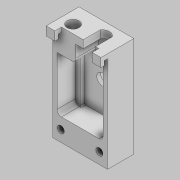
# Autodesk Inventor part: case
Saved by Autodesk Inventor 2021.4 (Build 254397000, 397)
## iProperties
Created: 2022-10-31
Part Number: case
Material: Generisch
Document SubType Name: Modeling
Designer: Tilman Preuschoff
Density: 1 g/cm^3
Appearance: Vorgabe
Author: Tilman Preuschoff
Autodesk Inventor part; units mm, degrees
ref_plane "YZ Plane" through (0, 0, 0) normal (1, 0, 0) x (0, 1, 0)
ref_plane "XZ Plane" through (0, 0, 0) normal (0, 1, 0) x (-1, 0, 0)
ref_plane "XY Plane" through (0, 0, 0) normal (0, 0, 1) x (1, 0, 0)
sketch "Skizze1" plane through (0, 0, 0) normal (0, 0, 1) x (1, 0, 0)
  line L0 (-12.5, 22.5) -> (12.5, 22.5)
  line L1 (12.5, 22.5) -> (12.5, -22.5)
  line L2 (12.5, -22.5) -> (-12.5, -22.5)
  line L3 (-12.5, -22.5) -> (-12.5, 22.5)
  line L4 (-12.5, 22.5) -> (12.5, -22.5) construction
  line L5 (12.5, 22.5) -> (-12.5, -22.5) construction
  point P0 (0, 0)
  dimension "d0" = 25
  dimension "d1" = 45
  constraints: 12 end point, 2 midpoint, 2 parallel, 1 horizontal, 1 perpendicular
  measures "d0" distance between parallel lines of L1 L3
  measures "d1" distance between parallel lines of L0 L2
extrude "Extrusion1" add sketch "Skizze1" along normal blind 12
sketch "Skizze2" plane through (0, 0, 12) normal (0, 0, 1) x (1, 0, 0)
  line L0 (-8.5, 19) -> (8.5, 19)
  line L1 (10.5, 17) -> (10.5, -11)
  line L2 (8.5, -13) -> (-8.5, -13)
  line L3 (-10.5, -11) -> (-10.5, 17)
  line L4 (-10.5, 19) -> (10.5, -13) construction
  line L5 (10.5, 19) -> (-10.5, -13) construction
  line L6 (12.5, 22.5) -> (-12.5, 22.5) projected
  arc A0 (-8.5, 19) -> (-10.5, 17) centre (-8.5, 17) ccw
  arc A1 (10.5, 17) -> (8.5, 19) centre (8.5, 17) ccw
  arc A2 (8.5, -13) -> (10.5, -11) centre (8.5, -11) ccw
  arc A3 (-10.5, -11) -> (-8.5, -13) centre (-8.5, -11) ccw
  point P0 (0, 0)
  point P1 (0, 3)
  point P2 (0, 3)
  dimension "d4" = 21
  dimension "d5" = 3.5
  dimension "d6" = 32
  dimension "d7" = 2
  constraints: 12 end point, 8 point on circle, 8 point on line, 8 tangent, 4 centre point, 3 equal radius, 3 midpoint, 2 parallel, 1 horizontal, 1 perpendicular, 1 vertical alignment
  measures "d4" distance between parallel lines of L1 L3
  measures "d5" distance between parallel lines of L6 L0
  measures "d6" distance between parallel lines of L2 L0
  measures "d7" radius of A0
extrude "Extrusion2" cut sketch "Skizze2" against normal blind 8.2
sketch "Skizze4" plane through (0, 0, 3.8) normal (0, 0, 1) x (1, 0, 0)
  line L0 (-12.5, -22.5) -> (12.5, -22.5) projected
  point P0 (0, 0)
  point P1 (0, 1)
  dimension "d79" = 23.5
  constraints: 1 vertical alignment
  measures "d79" distance from line of L0 point (0, 1)
hole "Bohrung2" at (0, 1, 3.8) direction (0, 0, -1) diameter 5.2 end through all
sketch "Skizze5" plane through (0, 0, 3.8) normal (0, 0, 1) x (1, 0, 0)
  line L0 (-8.5, 19) -> (8.5, 19) projected
  line L1 (-7.7, 19) -> (6.95, 19)
  line L2 (8.2, 21) -> (8.2, -12.5)
  line L3 (7.7, -13) -> (-7.7, -13)
  line L4 (-8.2, -12.5) -> (-8.2, 18.5)
  arc A0 (-7.7, 19) -> (-8.2, 18.5) centre (-7.7, 18.5) ccw
  arc A1 (7.7, -13) -> (8.2, -12.5) centre (7.7, -12.5) ccw
  arc A2 (-8.2, -12.5) -> (-7.7, -13) centre (-7.7, -12.5) ccw
  line L5 (10.5, 17) -> (10.5, -11) projected
  line L6 (6.95, 19) -> (7.7, 19)
  line L7 (8.2, 21) -> (8.2, 18.5)
  arc A3 (8.2, 18.5) -> (7.7, 19) centre (7.7, 18.5) ccw
  line L8 (-10.5, -11) -> (-10.5, 17) projected
  line L9 (8.5, -13) -> (-8.5, -13) projected
  point P0 (0, 0)
  point P1 (-8.2, 19)
  point P2 (8.2, 19)
  point P3 (8.2, 18.5)
  point P4 (4, -13)
  point P5 (7.7, -13)
  point P6 (6.2, 19)
  dimension "d28" = 0.5
  dimension "d29" = 2.3
  dimension "d39" = 0.5
  dimension "d67" = 0.5
  dimension "d73" = 2.3
  constraints: 12 end point, 8 point on circle, 8 tangent, 7 point on line, 4 centre point, 2 parallel, 2 perpendicular, 1 equal radius, 1 horizontal, 1 horizontal alignment
  measures "d28" radius of A0
  measures "d29" distance between parallel lines of L5 L2
  measures "d39" radius of A3
  measures "d67" radius of A1
  measures "d73" distance between parallel lines of L8 L4
sketch "Skizze6" plane through (0, 0, 12) normal (0, 0, 1) x (1, 0, 0)
  line L0 (12.5, 22.5) -> (-12.5, 22.5) projected
  line L1 (-8.5, 19) -> (8.5, 19) projected
  line L2 (-1.1, 22.5) -> (5.9, 22.5)
  line L3 (5.9, 22.5) -> (5.9, 19)
  line L4 (5.9, 19) -> (-1.1, 19)
  line L5 (-1.1, 19) -> (-1.1, 22.5)
  line L6 (12.5, -22.5) -> (12.5, 22.5) projected
  line L7 (7.95, 22) -> (7.95, 17) projected
  point P0 (0, 0)
  point P1 (6.95, 22)
  point P2 (8.5, 19)
  point P3 (5.9, 20.75)
  point P4 (7.95, 19.5)
  dimension "d34" = 7
  dimension "d38" = 6.6
  constraints: 8 end point, 2 midpoint, 2 parallel, 1 horizontal, 1 perpendicular, 1 point on line, 2 other
  measures "d34" distance between parallel lines of L3 L5
  measures "d38" distance between parallel lines of L6 L3
extrude "Extrusion4" [suppressed]
extrude "Extrusion5" cut sketch "Skizze5" against normal blind 2 contours L0 A3 L2 A1 L3 A2 L4 A0
sketch "Skizze7" plane through (-12.5, -22.5, 0) normal (0, -1, 0) x (1, 0, 0)
  line L0 (0, 0) -> (25, 0) projected
  point P0 (12.5, 0)
  point P1 (12.5, 7)
  point P2 (12.5, 0)
  dimension "d42" = 7
  constraints: 1 midpoint, 1 vertical alignment
  measures "d42" distance from line of point (12.5, 7) L0
hole "Bohrung3" at (0, -22.5, 7) direction (0, 1, 0) diameter 5.6 depth 8
sketch "Skizze11" plane through (-12.5, 22.5, 0) normal (0, 1, 0) x (1, 0, 0)
  line L0 (4, -12) -> (21, -12) projected
  line L1 (13.95, -12) -> (19.45, -12)
  line L2 (19.45, -12) -> (19.45, -4)
  line L3 (19.45, -4) -> (13.95, -4)
  line L4 (13.95, -4) -> (13.95, -12)
  line L5 (25, 0) -> (25, -12) projected
  line L6 (25, 0) -> (0, 0) projected
  circle A0 centre (16.7, -6.1) radius 3.3
  point P0 (12.5, 0)
  point P1 (7.5, -12)
  point P2 (16.7, -4)
  point P3 (19.45, -4.2759)
  point P4 (13.95, -4.2759)
  dimension "d68" = 5.5
  dimension "d69" = 5.55
  dimension "d91" = 6.6
  dimension "d92" = 6.1
  dimension "d93" = 8
  constraints: 8 end point, 2 parallel, 1 centre point, 1 horizontal, 1 midpoint, 1 perpendicular, 1 point on line, 1 vertical alignment
  measures "d68" distance between parallel lines of L2 L4
  measures "d69" distance between parallel lines of L5 L2
  measures "d91" diameter of A0
  measures "d92" distance from line of L6 A0.centre
  measures "d93" distance between parallel lines of L3 L0
extrude "Extrusion8" cut sketch "Skizze11" against normal up to surface (3.5 mm away) contours L4 A0 L2 L0 | L4 A0 L3 L2 | A0 L3
sketch "Skizze13" plane through (0, 0, 12) normal (0, 0, 1) x (1, 0, 0)
  line L0 (12.5, 22.5) -> (-12.5, 22.5) projected
  line L1 (-12.5, 22.5) -> (-2, 22.5)
  line L2 (-2, 22.5) -> (-2, 13.5)
  line L3 (-4, 11.5) -> (-12.5, 11.5)
  line L4 (-12.5, 11.5) -> (-12.5, 22.5)
  arc A0 (-4, 11.5) -> (-2, 13.5) centre (-4, 13.5) ccw
  point P0 (0, 0)
  dimension "d94" = 2
  dimension "d95" = 10.5
  dimension "d96" = 11
  constraints: 8 end point, 2 parallel, 2 point on circle, 2 tangent, 1 centre point, 1 horizontal, 1 perpendicular
  measures "d94" radius of A0
  measures "d95" distance between parallel lines of L4 L2
  measures "d96" distance from line of L1.end L3
extrude "Extrusion9" add sketch "Skizze13" against normal up to surface (12 mm away)
sketch "Skizze14" plane through (-12.5, 22.5, 0) normal (0, 1, 0) x (1, 0, 0)
  circle A0 centre (5.5, -8.25) radius 2.75
  line L0 (2, -3.8) -> (2, -12) projected
  line L1 (25, 0) -> (0, 0) projected
  line L2 (0, 0) -> (0, -12) projected
  point P0 (12.5, 0)
  point P1 (12.9295, 0.3417)
  point P2 (1.9355, -9.867)
  dimension "d101" = 5.5
  dimension "d102" = 8.25
  dimension "d114" = 5.5
  constraints: 1 centre point
  measures "d101" diameter of A0
  measures "d102" distance from line of L1 A0.centre
  measures "d114" distance from line of A0.centre L2
extrude "Extrusion10" cut sketch "Skizze14" against normal up to surface (11 mm away)
sketch "Skizze15" plane through (0, 0, 0) normal (0, 0, -1) x (-1, 0, 0)
  line L0 (-12.5, 22.5) -> (12.5, 22.5) projected
  line L1 (12.5, 22.5) -> (12.5, -22.5) projected
  point P0 (0, 0)
  point P1 (7, 16.5)
  point P2 (0, 0)
  dimension "d112" = 6
  dimension "d113" = 5.5
  constraints: 1 coincident
  measures "d112" distance from line of point (7, 16.5) L0
  measures "d113" distance from line of point (7, 16.5) L1
hole "Bohrung6" at (-7, 16.5, 0) direction (0, 0, 1) diameter 5.6 depth 8
sketch "Skizze20" plane through (-12.5, -22.5, 0) normal (0, -1, 0) x (1, 0, 0)
  line L0 (0, 12) -> (0.7, 12) projected
  line L1 (0, 0) -> (25, 0) projected
  line L2 (0, 12) -> (25, 12)
  line L3 (25, 12) -> (25, 0)
  line L4 (25, 0) -> (0, 0)
  line L5 (0, 0) -> (0, 12)
  circle A0 centre (12.5, 7) radius 2.8 projected
  circle A1 centre (12.5, 7) radius 2.8
  point P0 (12.5, 0)
  constraints: 8 end point, 2 parallel, 1 centre point, 1 coincident, 1 horizontal, 1 perpendicular
extrude "Extrusion15" add sketch "Skizze20" along normal blind 0.7
sketch "Skizze21" plane through (0, 0, 12) normal (0, 0, 1) x (1, 0, 0)
  line L0 (-12.5, 22.5) -> (-12.5, -23.2) projected
  line L1 (-12.5, 22.5) -> (-8.5, 22.5)
  line L2 (-8.5, 22.5) -> (-8.5, 20.5)
  line L3 (-8.5, 20.5) -> (-12.5, 20.5)
  line L4 (-12.5, 20.5) -> (-12.5, 22.5)
  line L5 (12.5, 22.5) -> (12.5, -23.2) projected
  line L6 (12.5, 22.5) -> (8.5, 22.5)
  line L7 (8.5, 22.5) -> (8.5, 20.5)
  line L8 (8.5, 20.5) -> (12.5, 20.5)
  line L9 (12.5, 20.5) -> (12.5, 22.5)
  point P0 (0, 0)
  dimension "d139" = 2
  dimension "d140" = 2
  dimension "d141" = 4
  dimension "d142" = 4
  constraints: 16 end point, 4 parallel, 2 horizontal, 2 perpendicular
  measures "d139" distance between parallel lines of L6 L8
  measures "d140" distance between parallel lines of L1 L3
  measures "d141" distance between parallel lines of L5 L7
  measures "d142" distance between parallel lines of L0 L2
extrude "Extrusion16" add sketch "Skizze21" along normal blind 1.5
sketch "Skizze22" plane through (0, 0, 13.5) normal (0, 0, 1) x (1, 0, 0)
  line L0 (-12.5, 22.5) -> (-12.5, -23.2) projected
  line L1 (8.5, 20.5) -> (8.5, 22.5) projected
  line L2 (12.5, 20.5) -> (12.5, -23.2) projected
  line L3 (8.5, 22.5) -> (12.5, 22.5)
  line L4 (12.5, 22.5) -> (12.5, 18.5)
  line L5 (12.5, 18.5) -> (8.5, 18.5)
  line L6 (8.5, 18.5) -> (8.5, 22.5)
  line L7 (-8.5, 22.5) -> (-8.5, 20.5) projected
  line L8 (-12.5, 20.5) -> (-12.5, -23.2) projected
  line L9 (-8.5, 22.5) -> (-12.5, 22.5)
  line L10 (-12.5, 22.5) -> (-12.5, 18.5)
  line L11 (-12.5, 18.5) -> (-8.5, 18.5)
  line L12 (-8.5, 18.5) -> (-8.5, 22.5)
  point P0 (0, 0)
  dimension "d145" = 4
  dimension "d146" = 4
  constraints: 16 end point, 4 parallel, 2 horizontal, 2 perpendicular, 2 point on line
  measures "d145" distance between parallel lines of L9 L11
  measures "d146" distance between parallel lines of L3 L5
extrude "Extrusion17" add sketch "Skizze22" along normal blind 1.5
sketch "Skizze23" plane through (0, 0, 12) normal (0, 0, 1) x (1, 0, 0)
  line L0 (-8.8, -18.1) -> (8.8, -18.1)
  line L1 (-12.5, 20.5) -> (-12.5, -23.2) projected
  line L2 (12.5, 20.5) -> (12.5, -23.2) projected
  line L3 (8.5, -13) -> (-8.5, -13) projected
  line L4 (12.5, -23.2) -> (-12.5, -23.2) projected
  point P0 (0, 0)
  dimension "d149" = 3.7
  dimension "d150" = 3.7
  dimension "d152" = 5.1
  dimension "d153" = 10.2
  constraints: 2 end point, 1 horizontal
  measures "d149" distance from line of L1 L0.start
  measures "d150" distance from line of L2 L0.end
  measures "d152" distance between parallel lines of L4 L0
  measures "d153" distance between parallel lines of L4 L3
hole "Bohrung7" at (-8.8, -18.1, 12) at (8.8, -18.1, 12) direction (0, 0, -1) diameter 3.2 depth 8
equation "\"d152\" = 0.5 * d153"
